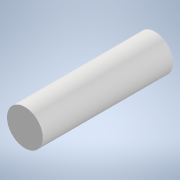
# Autodesk Inventor part: OdroidPlateSpacer
Saved by Autodesk Inventor 2020 (Build 240168000, 168)
## iProperties
Created: 2019-06-17
Part Number: OdroidPlateSpacer
Material: Generic
Document SubType Name: Modeling
Designer: amirt
Density: 1 g/cm^3
Appearance: Default
Author: amirt
Autodesk Inventor part; units mm, degrees
ref_plane "YZ Plane" through (0, 0, 0) normal (1, 0, 0) x (0, 1, 0)
ref_plane "XZ Plane" through (0, 0, 0) normal (0, 1, 0) x (-1, 0, 0)
sketch "Sketch2" plane through (0, 0, 0) normal (0, 0, 1) x (1, 0, 0)
  arc A0 (-66.5677, -26.035) -> (-67.8377, -24.765) centre (-67.8377, -26.035) ccw projected
  line L0 (-66.5677, -26.035) -> (-66.5677, -27.305) projected
  arc A1 (-67.8377, -28.575) -> (-66.5677, -27.305) centre (-67.8377, -27.305) ccw projected
  arc A2 (-66.5677, -51.435) -> (-67.8377, -50.165) centre (-67.8377, -51.435) ccw projected
  line L1 (-66.5677, -51.435) -> (-66.5677, -52.705) projected
  arc A3 (-67.8377, -53.975) -> (-66.5677, -52.705) centre (-67.8377, -52.705) ccw projected
  arc A4 (21.3481, -24.765) -> (20.0781, -26.035) centre (21.3481, -26.035) ccw projected
  line L2 (20.0781, -27.305) -> (20.0781, -26.035) projected
  arc A5 (20.0781, -27.305) -> (21.3481, -28.575) centre (21.3481, -27.305) ccw projected
  arc A6 (21.3481, -50.165) -> (20.0781, -51.435) centre (21.3481, -51.435) ccw projected
  line L3 (20.0781, -52.705) -> (20.0781, -51.435) projected
  arc A7 (20.0781, -52.705) -> (21.3481, -53.975) centre (21.3481, -52.705) ccw projected
  line L4 (21.3481, -24.765) -> (44.2081, -24.765) projected
  line L5 (44.2081, -28.575) -> (21.3481, -28.575) projected
  circle A8 centre (21.9831, -26.67) radius 1.905
  line L6 (-90.6977, -24.765) -> (-67.8377, -24.765)
  line L7 (-67.8377, -28.575) -> (-90.6977, -28.575)
  line L8 (-90.6977, -50.165) -> (-67.8377, -50.165)
  line L9 (-67.8377, -53.975) -> (-90.6977, -53.975)
  line L10 (21.3481, -50.165) -> (44.2081, -50.165)
  line L11 (44.2081, -53.975) -> (21.3481, -53.975)
  circle A9 centre (21.9831, -52.07) radius 1.905
  circle A10 centre (-68.4727, -52.07) radius 1.905
  circle A11 centre (-68.4727, -26.67) radius 1.905
  point P0 (0, 0)
  constraints: 12 end point, 12 tangent, 6 horizontal, 4 centre point, 12 other
ref_plane "Work Plane1" through (-61.5205, -96.6844, 13.8416) normal (0, 0, -1) x (0, 1, 0)
extrude "Extrusion1" add sketch "Sketch2" along normal up to surface (13.8416 mm away) contours A11 | A10 | A8 | A9
body "Solid1"
